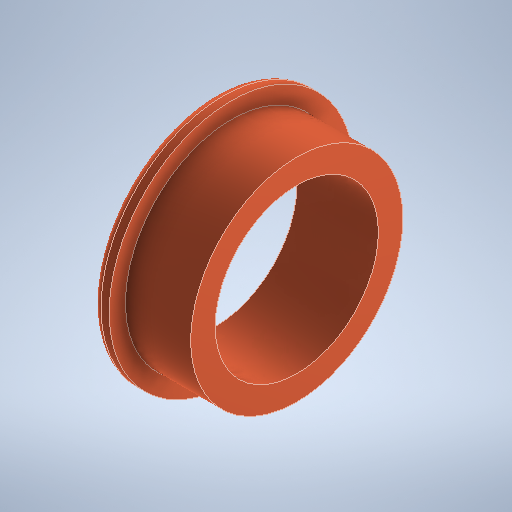
# Autodesk Inventor part: 101 part 3
Saved by Autodesk Inventor 2025.1 (Build 291241000, 241)
## iProperties
Created: 2024-09-02
Part Number: 101 part 3
Material: Copper, Alloy
Document SubType Name: Modeling
Designer: ffogue
Density: 8.92 g/cm^3
Appearance: Copper - Satin
Author: ffogue
Autodesk Inventor part; units mm, degrees
ref_plane "YZ Plane" through (0, 0, 0) normal (1, 0, 0) x (0, 1, 0)
ref_plane "XZ Plane" through (0, 0, 0) normal (0, 1, 0) x (-1, 0, 0)
ref_plane "XY Plane" through (0, 0, 0) normal (0, 0, 1) x (1, 0, 0)
sketch "Sketch1" plane through (0, 0, 0) normal (0, 0, 1) x (1, 0, 0)
  line L0 (0, 0) -> (0, 15)
  line L1 (0, 15) -> (2, 15)
  line L2 (2, 15) -> (2, 13)
  line L3 (2, 13) -> (10, 13)
  line L4 (10, 13) -> (10, 0)
  line L5 (10, 0) -> (0, 0)
  dimension "d0" = 2
  dimension "d1" = 8
  dimension "d2" = 30
  dimension "d3" = 26
  constraints: 12 end point, 5 perpendicular, 1 vertical
  measures "d0" distance of L0.end L1.end
  measures "d1" distance of L2.end L3.end
  measures "d2" diameter of L1 L5
  measures "d3" diameter of L3 L5
revolve "Revolution1" add sketch "Sketch1" angle 360 about axis through (10, 0, 0) along (-1, 0, 0)
fillet "Fillet1" radius 1 1 edges at (0, -15, 0)
sketch "Sketch2" plane through (10, 0, 0) normal (1, 0, 0) x (0, 0, -1)
  circle A0 centre (0, 0) radius 13 projected
  point P0 (0, 0)
  constraints: 1 coincident
hole "Hole1" at (10, 0, 0) direction (-1, 0, 0) diameter 20 depth 10
body "Solid1"
